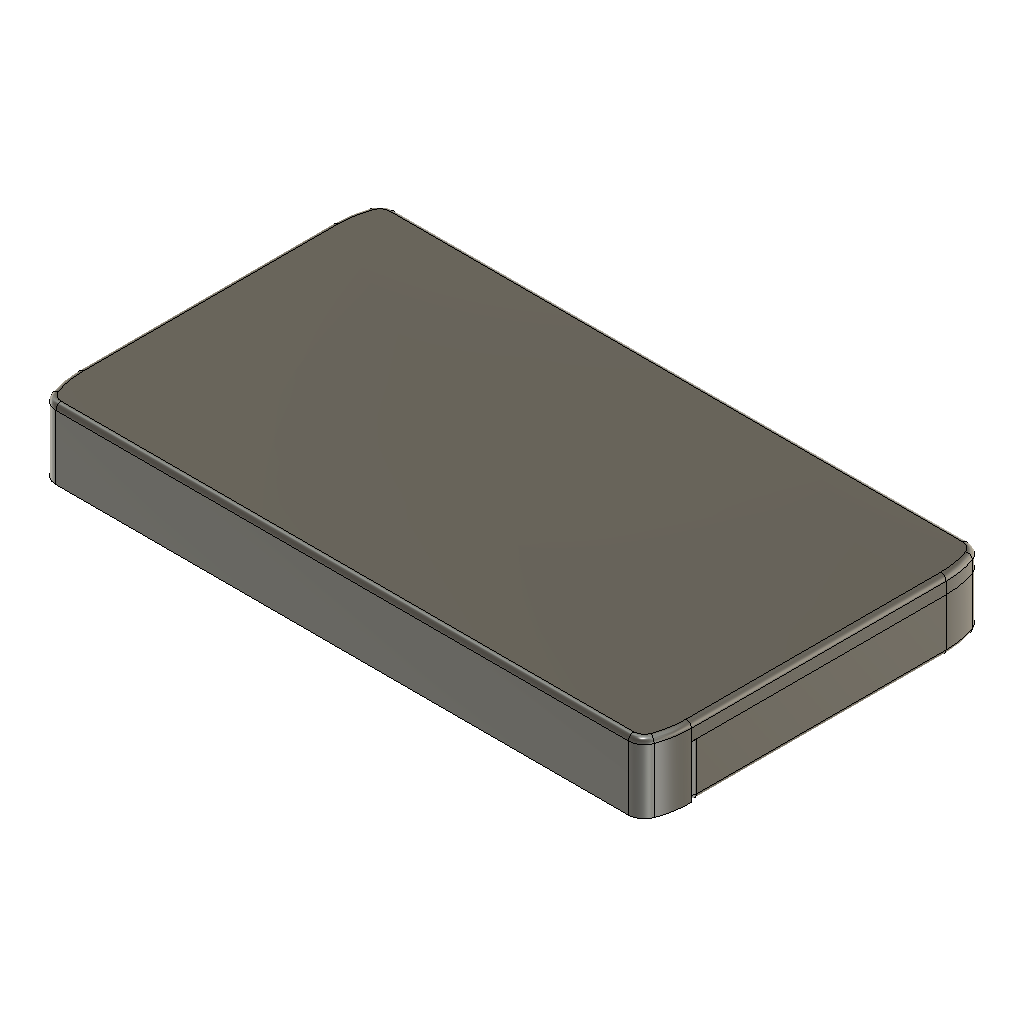
Card Wallet Var #1 (Autodesk Fusion 360 design; units mm, degrees)
part number: 2026-09-20-19-03-01-787
Autodesk Fusion 360 part; units mm, degrees
sketch "Sketch1" plane through (0, 0, 0) normal (0, 0, 1) x (1, 0, 0)
  line L0 (3, 0) -> (82.6, 0)
  line L1 (85.6, 3) -> (85.6, 50.98)
  line L2 (82.6, 53.98) -> (3, 53.98)
  line L3 (0, 50.98) -> (0, 3)
  arc A0 (3, 53.98) -> (0, 50.98) centre (3, 50.98) ccw
  arc A1 (85.6, 50.98) -> (82.6, 53.98) centre (82.6, 50.98) ccw
  arc A2 (82.6, 0) -> (85.6, 3) centre (82.6, 3) ccw
  arc A3 (0, 3) -> (3, 0) centre (3, 3) ccw
  arc A4 (-13.9706, 56.98) -> (-15, 50.98) centre (3, 50.98) ccw
  line L4 (-15, 50.98) -> (-15, 3)
  arc A5 (-15, 3) -> (-13.9706, -3) centre (3, 3) ccw
  arc A6 (99.5706, -3) -> (100.6, 3) centre (82.6, 3) ccw
  line L5 (100.6, 3) -> (100.6, 50.98)
  arc A7 (100.6, 50.98) -> (99.5706, 56.98) centre (82.6, 50.98) ccw
  line L6 (-11.1421, -5) -> (96.7421, -5)
  line L7 (96.7421, 58.98) -> (-11.1421, 58.98)
  arc A8 (-11.1421, 58.98) -> (-13.9706, 56.98) centre (-11.1421, 55.98) ccw
  arc A9 (99.5706, 56.98) -> (96.7421, 58.98) centre (96.7421, 55.98) ccw
  arc A10 (96.7421, -5) -> (99.5706, -3) centre (96.7421, -2) ccw
  arc A11 (-13.9706, -3) -> (-11.1421, -5) centre (-11.1421, -2) ccw
  point P0 (85.6, 0)
  point P1 (0, 53.98)
  dimension "d1" = 85.6
  dimension "d2" = 53.98
  dimension "d3" = 3
  dimension "d8" = 15
  dimension "d9" = 15
  dimension "d10" = 5
  dimension "d11" = 3
  dimension "d12" = 5
  constraint horizontal L0
  constraint vertical L1
  constraint horizontal L2
  constraint vertical L3
  constraint coincident P1 L2
  constraint coincident P1 L3
  constraint tangent L2 A0
  constraint tangent L3 A0
  constraint tangent L1 A1
  constraint tangent L2 A1
  constraint equal A0 A1
  constraint coincident P0 L0
  constraint coincident P0 L1
  constraint tangent L0 A2
  constraint tangent L1 A2
  constraint equal A0 A2
  constraint coincident origin L0
  constraint coincident origin L3
  constraint tangent L0 A3
  constraint tangent L3 A3
  constraint equal A0 A3
  constraint concentric A2 A6
  constraint concentric A1 A7
  constraint tangent A6 L5
  constraint tangent L5 A7
  constraint concentric A0 A4
  constraint concentric A3 A5
  constraint tangent A4 L4
  constraint tangent L4 A5
  constraint tangent L7 A8
  constraint tangent A4 A8
  constraint tangent L7 A9
  constraint tangent A7 A9
  constraint equal A8 A9
  constraint tangent A6 A10
  constraint tangent L6 A10
  constraint equal A8 A10
  constraint tangent L6 A11
  constraint tangent A5 A11
  constraint equal A8 A11
  measures "d1" distance of origin P0
  measures "d2" distance of origin P1
  measures "d3" radius of A0
  measures "d8" distance of L1 L5
  measures "d9" distance of L3 L4
  measures "d10" distance of L2 L7
  measures "d11" radius of A8
  measures "d12" distance of L0 L6
extrude "Extrude1" add sketch "Sketch1" along normal blind 1 contours L0 L1 L2 L3 A0 A1 A2 A3 | A4 L4 A5 A6 L5 A7 L6 L7 A8 A9 A10 A11 makes body 1
extrude "Extrude2" add sketch "Sketch1" along normal blind 10 separate body makes body 2
sketch "Sketch2" plane through (0, 0, 10) normal (0, 0, 1) x (-1, 0, 0)
  arc A0 (0, -3) -> (-3, 0) centre (-3, -3) ccw
  line L0 (0, -3) -> (0, -50.98)
  arc A1 (-3, -53.98) -> (0, -50.98) centre (-3, -50.98) ccw
  line L1 (-3, -53.98) -> (-82.6, -53.98)
  arc A2 (-85.6, -50.98) -> (-82.6, -53.98) centre (-82.6, -50.98) ccw
  line L2 (-85.6, -50.98) -> (-85.6, -3)
  arc A3 (-82.6, 0) -> (-85.6, -3) centre (-82.6, -3) ccw
  line L3 (-82.6, 0) -> (-3, 0)
  arc A4 (13.9706, 3) -> (11.1421, 5) centre (11.1421, 2) ccw
  line L4 (11.1421, 5) -> (-96.7421, 5)
  arc A5 (-96.7421, 5) -> (-99.5706, 3) centre (-96.7421, 2) ccw
  arc A6 (-99.5706, 3) -> (-100.6, -3) centre (-82.6, -3) ccw
  line L5 (-100.6, -3) -> (-100.6, -50.98)
  arc A7 (-100.6, -50.98) -> (-99.5706, -56.98) centre (-82.6, -50.98) ccw
  arc A8 (-99.5706, -56.98) -> (-96.7421, -58.98) centre (-96.7421, -55.98) ccw
  line L6 (-96.7421, -58.98) -> (11.1421, -58.98)
  arc A9 (11.1421, -58.98) -> (13.9706, -56.98) centre (11.1421, -55.98) ccw
  arc A10 (13.9706, -56.98) -> (15, -50.98) centre (-3, -50.98) ccw
  line L7 (15, -50.98) -> (15, -3)
  arc A11 (15, -3) -> (13.9706, 3) centre (-3, -3) ccw
  circle A12 centre (7.5, -5) radius 5.1
  circle A13 centre (-93.1, -48.98) radius 5.1
  arc A14 (13, -3) -> (12.0849, 2.3333) centre (-3, -3) ccw
  arc A15 (12.0849, 2.3333) -> (11.1421, 3) centre (11.1421, 2) ccw
  line L8 (11.1421, 3) -> (-96.7421, 3)
  arc A16 (-96.7421, 3) -> (-97.6849, 2.3333) centre (-96.7421, 2) ccw
  arc A17 (-97.6849, 2.3333) -> (-98.6, -3) centre (-82.6, -3) ccw
  line L9 (13, -3) -> (15, -3)
  line L10 (-98.6, -3) -> (-100.6, -3)
  dimension "d17" = 10.2
  dimension "d18" = 7.5
  dimension "d19" = 10
  dimension "d20" = 10.2
  dimension "d21" = 10
  dimension "d22" = 7.5
  dimension "d23" = -2
  constraint coincident L7.end A11.start
  constraint perpendicular L7 L9
  constraint coincident A6.end L5.start
  constraint perpendicular A6 L10
  measures "d17" diameter of A12
  measures "d18" distance of L0 A12.centre
  measures "d19" distance of L4 A12.centre
  measures "d20" diameter of A13
  measures "d21" distance of L6 A13.centre
  measures "d22" distance of L5 A13.centre
extrude "Extrude3" cut sketch "Sketch2" against normal blind 2.1 contours A4 L4 A5 A6 A11 A14 A15 L8 A16 A17 L9 L10 | A12 | A13 bodies 2
extrude "Extrude4" add sketch "Sketch2" along normal blind 2.2 separate body makes body 3
combine "Combine1" operation add target body 1 tool bodies 2
extrude "Extrude5" add sketch "Sketch2" against normal blind 9.9 contours A4 L4 A5 A6 A11 A14 A15 L8 A16 A17 L9 L10 bodies 3
sketch "Sketch3" plane through (0, 0, 12.2) normal (0, 0, 1) x (-1, 0, 0)
  circle A0 centre (-93.1, -48.98) radius 5.1
  circle A1 centre (7.5, -5) radius 5.1
  arc A2 (-85.6, -50.98) -> (-82.6, -53.98) centre (-82.6, -50.98) ccw
  line L0 (-85.6, -50.98) -> (-85.6, -3)
  arc A3 (-82.6, 0) -> (-85.6, -3) centre (-82.6, -3) ccw
  line L1 (-82.6, 0) -> (-3, 0)
  arc A4 (0, -3) -> (-3, 0) centre (-3, -3) ccw
  line L2 (0, -3) -> (0, -50.98)
  arc A5 (-3, -53.98) -> (0, -50.98) centre (-3, -50.98) ccw
  line L3 (-3, -53.98) -> (-82.6, -53.98)
  arc A6 (15, -3) -> (13.9706, 3) centre (-3, -3) ccw
  arc A7 (13.9706, 3) -> (11.1421, 5) centre (11.1421, 2) ccw
  line L4 (11.1421, 5) -> (-96.7421, 5)
  arc A8 (-96.7421, 5) -> (-99.5706, 3) centre (-96.7421, 2) ccw
  arc A9 (-99.5706, 3) -> (-100.6, -3) centre (-82.6, -3) ccw
  line L5 (-100.6, -3) -> (-100.6, -50.98)
  arc A10 (-100.6, -50.98) -> (-99.5706, -56.98) centre (-82.6, -50.98) ccw
  arc A11 (-99.5706, -56.98) -> (-96.7421, -58.98) centre (-96.7421, -55.98) ccw
  line L6 (-96.7421, -58.98) -> (11.1421, -58.98)
  arc A12 (11.1421, -58.98) -> (13.9706, -56.98) centre (11.1421, -55.98) ccw
  arc A13 (13.9706, -56.98) -> (15, -50.98) centre (-3, -50.98) ccw
  line L7 (15, -50.98) -> (15, -3)
extrude "Extrude6" add sketch "Sketch3" along normal blind 1 contours A0 | A1 | A2 L0 A3 L1 A4 L2 A5 L3 | A6 A7 L4 A8 A9 L5 A10 A11 L6 A12 A13 L7 bodies 3
fillet "Fillet2" radius 1 1 faces at (62.0667, 18.9933, 13.2) on bodies 3
fillet "Fillet3" radius 1 1 faces at (62.0667, 18.9933, 0) on bodies 1
sketch "Sketch4" plane through (0, 0, 10) normal (0, 0, -1) x (1, 0, 0)
  line L0 (100.6, -3) -> (98.6, -3)
  arc A0 (98.6, -3) -> (97.6849, 2.3333) centre (82.6, -3) ccw
  arc A1 (97.6849, 2.3333) -> (96.7421, 3) centre (96.7421, 2) ccw
  line L1 (96.7421, 3) -> (-11.1421, 3)
  arc A2 (-11.1421, 3) -> (-12.0849, 2.3333) centre (-11.1421, 2) ccw
  arc A3 (-12.0849, 2.3333) -> (-13, -3) centre (3, -3) ccw
  line L2 (-13, -3) -> (-15, -3)
  line L3 (-15, -3) -> (-15, -50.98)
  arc A4 (-15, -50.98) -> (-13.9706, -56.98) centre (3, -50.98) ccw
  arc A5 (-13.9706, -56.98) -> (-11.1421, -58.98) centre (-11.1421, -55.98) ccw
  line L4 (-11.1421, -58.98) -> (96.7421, -58.98)
  arc A6 (96.7421, -58.98) -> (99.5706, -56.98) centre (96.7421, -55.98) ccw
  arc A7 (99.5706, -56.98) -> (100.6, -50.98) centre (82.6, -50.98) ccw
  line L5 (100.6, -50.98) -> (100.6, -3)
  circle A8 centre (-7.5, -5) radius 5.1
  circle A9 centre (93.1, -48.98) radius 5.1
  arc A10 (82.6, -53.98) -> (85.6, -50.98) centre (82.6, -50.98) ccw
  line L6 (82.6, -53.98) -> (3, -53.98)
  arc A11 (0, -50.98) -> (3, -53.98) centre (3, -50.98) ccw
  line L7 (0, -50.98) -> (0, -3)
  arc A12 (3, 0) -> (0, -3) centre (3, -3) ccw
  line L8 (3, 0) -> (82.6, 0)
  arc A13 (85.6, -3) -> (82.6, 0) centre (82.6, -3) ccw
  line L9 (85.6, -3) -> (85.6, -50.98)
extrude "Extrude7" add sketch "Sketch4" against normal blind 0.1 contours A8 | A9 bodies 3
sketch "Sketch7" plane through (0, 0, 10) normal (0, 0, 1) x (-1, 0, 0)
  line L0 (15, -3) -> (13, -3)
  arc A0 (13, -3) -> (12.0849, 2.3333) centre (-3, -3) ccw
  arc A1 (12.0849, 2.3333) -> (11.1421, 3) centre (11.1421, 2) ccw
  line L1 (11.1421, 3) -> (-96.7421, 3)
  arc A2 (-96.7421, 3) -> (-97.6849, 2.3333) centre (-96.7421, 2) ccw
  arc A3 (-97.6849, 2.3333) -> (-98.6, -3) centre (-82.6, -3) ccw
  line L2 (-98.6, -3) -> (-100.6, -3)
  line L3 (-100.6, -3) -> (-100.6, -50.98)
  arc A4 (-100.6, -50.98) -> (-99.5706, -56.98) centre (-82.6, -50.98) ccw
  arc A5 (-99.5706, -56.98) -> (-96.7421, -58.98) centre (-96.7421, -55.98) ccw
  line L4 (-96.7421, -58.98) -> (11.1421, -58.98)
  arc A6 (11.1421, -58.98) -> (13.9706, -56.98) centre (11.1421, -55.98) ccw
  arc A7 (13.9706, -56.98) -> (15, -50.98) centre (-3, -50.98) ccw
  line L5 (15, -50.98) -> (15, -3)
  arc A8 (0, -3) -> (-3, 0) centre (-3, -3) ccw
  line L6 (0, -3) -> (0, -50.98)
  arc A9 (-3, -53.98) -> (0, -50.98) centre (-3, -50.98) ccw
  line L7 (-3, -53.98) -> (-82.6, -53.98)
  arc A10 (-85.6, -50.98) -> (-82.6, -53.98) centre (-82.6, -50.98) ccw
  line L8 (-85.6, -50.98) -> (-85.6, -3)
  arc A11 (-82.6, 0) -> (-85.6, -3) centre (-82.6, -3) ccw
  line L9 (-82.6, 0) -> (-3, 0)
  circle A12 centre (7.5, -5) radius 5.1
  circle A13 centre (-93.1, -48.98) radius 5.1
  circle A14 centre (7.5, -5) radius 5.1
  circle A15 centre (-93.1, -48.98) radius 5.1
extrude "Extrude8" add sketch "Sketch7" against normal blind 0.1 contours A12 A14 | A13 A15 bodies 1
move_face "OffsetFaces1" offset -10 1 faces at (60.7807, -4.3333, 7.9) on bodies 1
sketch "Sketch8" plane through (0, 0, 10) normal (0, 0, 1) x (-1, 0, 0)
  line L0 (15, -3) -> (13, -3)
  arc A0 (13, -3) -> (12.0849, 2.3333) centre (-3, -3) ccw
  arc A1 (12.0849, 2.3333) -> (11.1421, 3) centre (11.1421, 2) ccw
  line L1 (11.1421, 3) -> (-96.7421, 3)
  arc A2 (-96.7421, 3) -> (-97.6849, 2.3333) centre (-96.7421, 2) ccw
  arc A3 (-97.6849, 2.3333) -> (-98.6, -3) centre (-82.6, -3) ccw
  line L2 (-98.6, -3) -> (-100.6, -3)
  line L3 (-100.6, -3) -> (-100.6, -50.98)
  arc A4 (-100.6, -50.98) -> (-99.5706, -56.98) centre (-82.6, -50.98) ccw
  arc A5 (-99.5706, -56.98) -> (-96.7421, -58.98) centre (-96.7421, -55.98) ccw
  line L4 (-96.7421, -58.98) -> (11.1421, -58.98)
  arc A6 (11.1421, -58.98) -> (13.9706, -56.98) centre (11.1421, -55.98) ccw
  arc A7 (13.9706, -56.98) -> (15, -50.98) centre (-3, -50.98) ccw
  line L5 (15, -50.98) -> (15, -3)
  arc A8 (0, -3) -> (-3, 0) centre (-3, -3) ccw
  line L6 (0, -3) -> (0, -50.98)
  arc A9 (-3, -53.98) -> (0, -50.98) centre (-3, -50.98) ccw
  line L7 (-3, -53.98) -> (-82.6, -53.98)
  arc A10 (-85.6, -50.98) -> (-82.6, -53.98) centre (-82.6, -50.98) ccw
  line L8 (-85.6, -50.98) -> (-85.6, -3)
  arc A11 (-82.6, 0) -> (-85.6, -3) centre (-82.6, -3) ccw
  line L9 (-82.6, 0) -> (-3, 0)
  line L10 (-78.8, -3.5) -> (-6.8, -3.5)
  line L11 (-6.8, -3.5) -> (-6.8, 6.5)
  line L12 (-6.8, 6.5) -> (-78.8, 6.5)
  line L13 (-78.8, 6.5) -> (-78.8, -3.5)
  line L14 (-78.8, -3.5) -> (-6.8, 6.5) construction
  line L15 (-6.8, -3.5) -> (-78.8, 6.5) construction
  point P0 (-42.8, 1.5)
  dimension "d43" = 1.5
  dimension "d44" = 42.8
  constraint horizontal L10
  constraint perpendicular L10 L11
  constraint parallel L10 L12
  constraint parallel L11 L13
  constraint coincident L14 P0
  constraint coincident L15 P0
  measures "d43" distance of L1 P0
  measures "d44" distance of L6 P0
extrude "Extrude9" cut sketch "Sketch8" against normal blind 9 contours L1 L9 L11 L13 bodies 1
fillet "Fillet4" radius 1 3 edges at (99.1, 3, 0) (100.3071, 3, 0.2929) (100.6, 3, 5.5) on bodies 1
equation "d18 = ( 15 / 2 ) * 1 mm"
equation "d22 = ( 15 / 2 ) * 1 mm"
equation "d44 = ( 85.6 / 2 ) * 1 mm"
